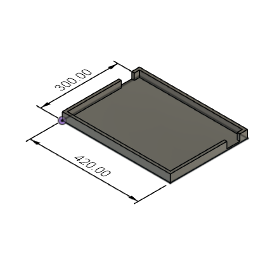
BasicMotorShell v3 (Autodesk Fusion 360 design; units mm, degrees)
Autodesk Fusion 360 part; units mm, degrees
sketch "BoxSketch" plane through (0, 0, 0) normal (0, 0, 1) x (1, 0, 0)
  line L0 (0, 0) -> (420, 0)
  line L1 (420, 0) -> (420, 300)
  line L2 (420, 300) -> (0, 300)
  line L3 (0, 300) -> (0, 0)
  dimension "d1" = 420
  dimension "d2" = 300
  constraint horizontal L0
  constraint vertical L1
  constraint horizontal L2
  constraint vertical L3
  constraint coincident L0.start L3.end
  measures "d1" distance of L0.start L0.end
  measures "d2" distance of L0.start L2.end
extrude "Extrude2" add sketch "BoxSketch" along normal blind 30
shell "Shell2" thickness 10 removed faces 1 at (140, 200, 30)
sketch "Sketch4" plane through (0, 0, 10) normal (0, 0, 1) x (-1, 0, 0)
  line L0 (-10, -290) -> (-10, -10)
  line L1 (-10, -10) -> (-410, -10)
  line L2 (-410, -10) -> (-410, -290)
  line L3 (-410, -290) -> (-10, -290)
  line L4 (-410, -10) -> (-10, -10)
  line L5 (-10, -10) -> (-10, -290)
  line L6 (-10, -290) -> (-410, -290)
  line L7 (-410, -290) -> (-410, -10)
  constraint horizontal L4
  constraint vertical L5
  constraint horizontal L6
  constraint vertical L7
  constraint coincident L0.start L3.end
  constraint coincident L1.end L2.start
extrude "Extrude7" cut sketch "Sketch4" against normal blind 5
sketch "MotorHoles" plane through (0, 0, 0) normal (-1, 0, 0) x (0, -1, 0)
  line L0 (-300, 0) -> (0, 0)
  line L1 (0, 0) -> (0, 30)
  line L2 (0, 30) -> (-300, 30)
  line L3 (-300, 30) -> (-300, 0)
  line L4 (-270, 35) -> (-220, 35)
  line L5 (-220, 35) -> (-220, 5)
  line L6 (-220, 5) -> (-270, 5)
  line L7 (-270, 5) -> (-270, 35)
  line L8 (-300, 0) -> (0, 0)
  dimension "d18" = 50
  dimension "d19" = 30
  dimension "d20" = 5
  dimension "d21" = 30
  constraint horizontal L4
  constraint vertical L5
  constraint horizontal L6
  constraint vertical L7
  measures "d18" distance of L5 L7
  measures "d19" distance of L3 L7
  measures "d20" distance of L6 L8
  measures "d21" distance of L4.end L5.end
extrude "Extrude8" cut sketch "MotorHoles" against normal blind 450 contours L2 L5 L6 L7
